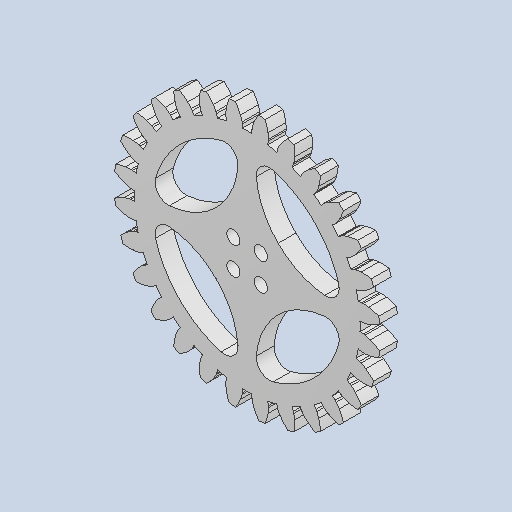
# Autodesk Inventor part: 最終段m2z28t4
Saved by Autodesk Inventor 2023 (Build 270158030, 158C)
## iProperties
Created: 2022-01-10
Part Number: 最終段m2z28t4
Material: Aluminum 2014-T6
Document SubType Name: Modeling
Designer: acps
Density: 2.78927 g/cm^3
Appearance: Satin
Author: acps
Autodesk Inventor part; units mm, degrees
ref_plane "YZ Plane" through (0, 0, 0) normal (1, 0, 0) x (0, 1, 0)
ref_plane "XZ Plane" through (0, 0, 0) normal (0, 1, 0) x (-1, 0, 0)
ref_plane "XY Plane" through (0, 0, 0) normal (0, 0, 1) x (1, 0, 0)
sketch "Sketch1" plane through (0, 0, 0) normal (0, 0, 1) x (1, 0, 0)
  arc A0 (1.1408, 26.6584) -> (1.0836, 26.2891) centre (3.5659, 26.0938) ccw
  arc A1 (1.5089, 27.8103) -> (1.1408, 26.6584) centre (7.8128, 25.1608) ccw
  arc A2 (2.6316, 29.8844) -> (1.5089, 27.8103) centre (12.3866, 23.2633) ccw
  arc A3 (-4.8199, 26.2439) -> (-4.7934, 25.8711) centre (-2.3299, 26.2331) ccw
  arc A4 (-4.7173, 27.4488) -> (-4.8199, 26.2439) centre (2.0181, 26.2684) ccw
  arc A5 (-4.0843, 29.7207) -> (-4.7173, 27.4488) centre (6.8995, 25.4363) ccw
  arc A6 (-10.5388, 24.5133) -> (-10.4301, 24.1558) centre (-8.1089, 25.0569) ccw
  arc A7 (-10.7069, 25.7109) -> (-10.5388, 24.5133) centre (-3.8778, 26.0589) ccw
  arc A8 (-10.5954, 28.0667) -> (-10.7069, 25.7109) centre (1.0664, 26.3339) ccw
  arc A9 (-15.7293, 21.5536) -> (-15.5438, 21.2292) centre (-13.4813, 22.6243) ccw
  arc A10 (-16.1597, 22.6838) -> (-15.7293, 21.5536) centre (-9.5792, 24.5427) ccw
  arc A11 (-16.5751, 25.0053) -> (-16.1597, 22.6838) centre (-4.8202, 25.9109) ccw
  arc A12 (-20.1311, 17.5131) -> (-19.878, 17.2382) centre (-18.1776, 19.0572) ccw
  arc A13 (-20.8022, 18.5192) -> (-20.1311, 17.5131) centre (-14.8003, 21.7958) ccw
  arc A14 (-21.7238, 20.69) -> (-20.8022, 18.5192) centre (-10.4651, 24.1887) ccw
  arc A15 (-23.5234, 12.5944) -> (-23.2155, 12.3827) centre (-21.9625, 14.5345) ccw
  arc A16 (-24.4015, 13.4259) -> (-23.5234, 12.5944) centre (-19.2792, 17.9559) ccw
  arc A17 (-25.7831, 15.3373) -> (-24.4015, 13.4259) centre (-15.5852, 21.2535) ccw
  arc A18 (-25.7362, 7.0442) -> (-25.3888, 6.9063) centre (-24.6461, 9.283) ccw
  arc A19 (-26.7773, 7.6595) -> (-25.7362, 7.0442) centre (-22.7914, 13.2157) ccw
  arc A20 (-28.5495, 9.2155) -> (-26.7773, 7.6595) centre (-19.9238, 17.2526) ccw
  arc A21 (-26.6584, 1.1408) -> (-26.2891, 1.0836) centre (-26.0938, 3.5659) ccw
  arc A22 (-27.8103, 1.5089) -> (-26.6584, 1.1408) centre (-25.1608, 7.8128) ccw
  arc A23 (-29.8844, 2.6316) -> (-27.8103, 1.5089) centre (-23.2633, 12.3866) ccw
  arc A24 (-26.2439, -4.8199) -> (-25.8711, -4.7934) centre (-26.2331, -2.3299) ccw
  arc A25 (-27.4488, -4.7173) -> (-26.2439, -4.8199) centre (-26.2684, 2.0181) ccw
  arc A26 (-29.7207, -4.0843) -> (-27.4488, -4.7173) centre (-25.4363, 6.8995) ccw
  arc A27 (-24.5133, -10.5388) -> (-24.1558, -10.4301) centre (-25.0569, -8.1089) ccw
  arc A28 (-25.7109, -10.7069) -> (-24.5133, -10.5388) centre (-26.0589, -3.8778) ccw
  arc A29 (-28.0667, -10.5954) -> (-25.7109, -10.7069) centre (-26.3339, 1.0664) ccw
  arc A30 (-21.5536, -15.7293) -> (-21.2292, -15.5438) centre (-22.6243, -13.4813) ccw
  arc A31 (-22.6838, -16.1597) -> (-21.5536, -15.7293) centre (-24.5427, -9.5792) ccw
  arc A32 (-25.0053, -16.5751) -> (-22.6838, -16.1597) centre (-25.9109, -4.8202) ccw
  arc A33 (-17.5131, -20.1311) -> (-17.2382, -19.878) centre (-19.0572, -18.1776) ccw
  arc A34 (-18.5192, -20.8022) -> (-17.5131, -20.1311) centre (-21.7958, -14.8003) ccw
  arc A35 (-20.69, -21.7238) -> (-18.5192, -20.8022) centre (-24.1887, -10.4651) ccw
  arc A36 (-12.5944, -23.5234) -> (-12.3827, -23.2155) centre (-14.5345, -21.9625) ccw
  arc A37 (-13.4259, -24.4015) -> (-12.5944, -23.5234) centre (-17.9559, -19.2792) ccw
  arc A38 (-15.3373, -25.7831) -> (-13.4259, -24.4015) centre (-21.2535, -15.5852) ccw
  arc A39 (-7.0442, -25.7362) -> (-6.9063, -25.3888) centre (-9.283, -24.6461) ccw
  arc A40 (-7.6595, -26.7773) -> (-7.0442, -25.7362) centre (-13.2157, -22.7914) ccw
  arc A41 (-9.2155, -28.5495) -> (-7.6595, -26.7773) centre (-17.2526, -19.9238) ccw
  arc A42 (-1.1408, -26.6584) -> (-1.0836, -26.2891) centre (-3.5659, -26.0938) ccw
  arc A43 (-1.5089, -27.8103) -> (-1.1408, -26.6584) centre (-7.8128, -25.1608) ccw
  arc A44 (-2.6316, -29.8844) -> (-1.5089, -27.8103) centre (-12.3866, -23.2633) ccw
  arc A45 (4.8199, -26.2439) -> (4.7934, -25.8711) centre (2.3299, -26.2331) ccw
  arc A46 (4.7173, -27.4488) -> (4.8199, -26.2439) centre (-2.0181, -26.2684) ccw
  arc A47 (4.0843, -29.7207) -> (4.7173, -27.4488) centre (-6.8995, -25.4363) ccw
  arc A48 (10.5388, -24.5133) -> (10.4301, -24.1558) centre (8.1089, -25.0569) ccw
  arc A49 (10.7069, -25.7109) -> (10.5388, -24.5133) centre (3.8778, -26.0589) ccw
  arc A50 (10.5954, -28.0667) -> (10.7069, -25.7109) centre (-1.0664, -26.3339) ccw
  arc A51 (15.7293, -21.5536) -> (15.5438, -21.2292) centre (13.4813, -22.6243) ccw
  arc A52 (16.1597, -22.6838) -> (15.7293, -21.5536) centre (9.5792, -24.5427) ccw
  arc A53 (16.5751, -25.0053) -> (16.1597, -22.6838) centre (4.8202, -25.9109) ccw
  arc A54 (20.1311, -17.5131) -> (19.878, -17.2382) centre (18.1776, -19.0572) ccw
  arc A55 (20.8022, -18.5192) -> (20.1311, -17.5131) centre (14.8003, -21.7958) ccw
  arc A56 (21.7238, -20.69) -> (20.8022, -18.5192) centre (10.4651, -24.1887) ccw
  arc A57 (23.5234, -12.5944) -> (23.2155, -12.3827) centre (21.9625, -14.5345) ccw
  arc A58 (24.4015, -13.4259) -> (23.5234, -12.5944) centre (19.2792, -17.9559) ccw
  arc A59 (25.7831, -15.3373) -> (24.4015, -13.4259) centre (15.5852, -21.2535) ccw
  arc A60 (25.7362, -7.0442) -> (25.3888, -6.9063) centre (24.6461, -9.283) ccw
  arc A61 (26.7773, -7.6595) -> (25.7362, -7.0442) centre (22.7914, -13.2157) ccw
  arc A62 (28.5495, -9.2155) -> (26.7773, -7.6595) centre (19.9238, -17.2526) ccw
  arc A63 (26.6584, -1.1408) -> (26.2891, -1.0836) centre (26.0938, -3.5659) ccw
  arc A64 (27.8103, -1.5089) -> (26.6584, -1.1408) centre (25.1608, -7.8128) ccw
  arc A65 (29.8844, -2.6316) -> (27.8103, -1.5089) centre (23.2633, -12.3866) ccw
  arc A66 (26.2439, 4.8199) -> (25.8711, 4.7934) centre (26.2331, 2.3299) ccw
  arc A67 (27.4488, 4.7173) -> (26.2439, 4.8199) centre (26.2684, -2.0181) ccw
  arc A68 (29.7207, 4.0843) -> (27.4488, 4.7173) centre (25.4363, -6.8995) ccw
  arc A69 (24.5133, 10.5388) -> (24.1558, 10.4301) centre (25.0569, 8.1089) ccw
  arc A70 (25.7109, 10.7069) -> (24.5133, 10.5388) centre (26.0589, 3.8778) ccw
  arc A71 (28.0667, 10.5954) -> (25.7109, 10.7069) centre (26.3339, -1.0664) ccw
  arc A72 (21.5536, 15.7293) -> (21.2292, 15.5438) centre (22.6243, 13.4813) ccw
  arc A73 (22.6838, 16.1597) -> (21.5536, 15.7293) centre (24.5427, 9.5792) ccw
  arc A74 (25.0053, 16.5751) -> (22.6838, 16.1597) centre (25.9109, 4.8202) ccw
  arc A75 (17.5131, 20.1311) -> (17.2382, 19.878) centre (19.0572, 18.1776) ccw
  arc A76 (18.5192, 20.8022) -> (17.5131, 20.1311) centre (21.7958, 14.8003) ccw
  arc A77 (20.69, 21.7238) -> (18.5192, 20.8022) centre (24.1887, 10.4651) ccw
  arc A78 (12.5944, 23.5234) -> (12.3827, 23.2155) centre (14.5345, 21.9625) ccw
  arc A79 (13.4259, 24.4015) -> (12.5944, 23.5234) centre (17.9559, 19.2792) ccw
  arc A80 (15.3373, 25.7831) -> (13.4259, 24.4015) centre (21.2535, 15.5852) ccw
  arc A81 (7.0442, 25.7362) -> (6.9063, 25.3888) centre (9.283, 24.6461) ccw
  arc A82 (7.6595, 26.7773) -> (7.0442, 25.7362) centre (13.2157, 22.7914) ccw
  arc A83 (9.2155, 28.5495) -> (7.6595, 26.7773) centre (17.2526, 19.9238) ccw
  arc A84 (-1.0836, 26.2891) -> (-1.1408, 26.6584) centre (-3.5659, 26.0938) ccw
  arc A85 (-1.1408, 26.6584) -> (-1.5089, 27.8103) centre (-7.8128, 25.1608) ccw
  arc A86 (-1.5089, 27.8103) -> (-2.6316, 29.8844) centre (-12.3866, 23.2633) ccw
  arc A87 (-6.9063, 25.3888) -> (-7.0442, 25.7362) centre (-9.283, 24.6461) ccw
  arc A88 (-7.0442, 25.7362) -> (-7.6595, 26.7773) centre (-13.2157, 22.7914) ccw
  arc A89 (-7.6595, 26.7773) -> (-9.2155, 28.5495) centre (-17.2526, 19.9238) ccw
  arc A90 (-12.3827, 23.2155) -> (-12.5944, 23.5234) centre (-14.5345, 21.9625) ccw
  arc A91 (-12.5944, 23.5234) -> (-13.4259, 24.4015) centre (-17.9559, 19.2792) ccw
  arc A92 (-13.4259, 24.4015) -> (-15.3373, 25.7831) centre (-21.2535, 15.5852) ccw
  arc A93 (-17.2382, 19.878) -> (-17.5131, 20.1311) centre (-19.0572, 18.1776) ccw
  arc A94 (-17.5131, 20.1311) -> (-18.5192, 20.8022) centre (-21.7958, 14.8003) ccw
  arc A95 (-18.5192, 20.8022) -> (-20.69, 21.7238) centre (-24.1887, 10.4651) ccw
  arc A96 (-21.2292, 15.5438) -> (-21.5536, 15.7293) centre (-22.6243, 13.4813) ccw
  arc A97 (-21.5536, 15.7293) -> (-22.6838, 16.1597) centre (-24.5427, 9.5792) ccw
  arc A98 (-22.6838, 16.1597) -> (-25.0053, 16.5751) centre (-25.9109, 4.8202) ccw
  arc A99 (-24.1558, 10.4301) -> (-24.5133, 10.5388) centre (-25.0569, 8.1089) ccw
  arc A100 (-24.5133, 10.5388) -> (-25.7109, 10.7069) centre (-26.0589, 3.8778) ccw
  arc A101 (-25.7109, 10.7069) -> (-28.0667, 10.5954) centre (-26.3339, -1.0664) ccw
  arc A102 (-25.8711, 4.7934) -> (-26.2439, 4.8199) centre (-26.2331, 2.3299) ccw
  arc A103 (-26.2439, 4.8199) -> (-27.4488, 4.7173) centre (-26.2684, -2.0181) ccw
  arc A104 (-27.4488, 4.7173) -> (-29.7207, 4.0843) centre (-25.4363, -6.8995) ccw
  arc A105 (-26.2891, -1.0836) -> (-26.6584, -1.1408) centre (-26.0938, -3.5659) ccw
  arc A106 (-26.6584, -1.1408) -> (-27.8103, -1.5089) centre (-25.1608, -7.8128) ccw
  arc A107 (-27.8103, -1.5089) -> (-29.8844, -2.6316) centre (-23.2633, -12.3866) ccw
  arc A108 (-25.3888, -6.9063) -> (-25.7362, -7.0442) centre (-24.6461, -9.283) ccw
  arc A109 (-25.7362, -7.0442) -> (-26.7773, -7.6595) centre (-22.7914, -13.2157) ccw
  arc A110 (-26.7773, -7.6595) -> (-28.5495, -9.2155) centre (-19.9238, -17.2526) ccw
  arc A111 (-23.2155, -12.3827) -> (-23.5234, -12.5944) centre (-21.9625, -14.5345) ccw
  arc A112 (-23.5234, -12.5944) -> (-24.4015, -13.4259) centre (-19.2792, -17.9559) ccw
  arc A113 (-24.4015, -13.4259) -> (-25.7831, -15.3373) centre (-15.5852, -21.2535) ccw
  arc A114 (-19.878, -17.2382) -> (-20.1311, -17.5131) centre (-18.1776, -19.0572) ccw
  arc A115 (-20.1311, -17.5131) -> (-20.8022, -18.5192) centre (-14.8003, -21.7958) ccw
  arc A116 (-20.8022, -18.5192) -> (-21.7238, -20.69) centre (-10.4651, -24.1887) ccw
  arc A117 (-15.5438, -21.2292) -> (-15.7293, -21.5536) centre (-13.4813, -22.6243) ccw
  arc A118 (-15.7293, -21.5536) -> (-16.1597, -22.6838) centre (-9.5792, -24.5427) ccw
  arc A119 (-16.1597, -22.6838) -> (-16.5751, -25.0053) centre (-4.8202, -25.9109) ccw
  arc A120 (-10.4301, -24.1558) -> (-10.5388, -24.5133) centre (-8.1089, -25.0569) ccw
  arc A121 (-10.5388, -24.5133) -> (-10.7069, -25.7109) centre (-3.8778, -26.0589) ccw
  arc A122 (-10.7069, -25.7109) -> (-10.5954, -28.0667) centre (1.0664, -26.3339) ccw
  arc A123 (-4.7934, -25.8711) -> (-4.8199, -26.2439) centre (-2.3299, -26.2331) ccw
  arc A124 (-4.8199, -26.2439) -> (-4.7173, -27.4488) centre (2.0181, -26.2684) ccw
  arc A125 (-4.7173, -27.4488) -> (-4.0843, -29.7207) centre (6.8995, -25.4363) ccw
  arc A126 (1.0836, -26.2891) -> (1.1408, -26.6584) centre (3.5659, -26.0938) ccw
  arc A127 (1.1408, -26.6584) -> (1.5089, -27.8103) centre (7.8128, -25.1608) ccw
  arc A128 (1.5089, -27.8103) -> (2.6316, -29.8844) centre (12.3866, -23.2633) ccw
  arc A129 (6.9063, -25.3888) -> (7.0442, -25.7362) centre (9.283, -24.6461) ccw
  arc A130 (7.0442, -25.7362) -> (7.6595, -26.7773) centre (13.2157, -22.7914) ccw
  arc A131 (7.6595, -26.7773) -> (9.2155, -28.5495) centre (17.2526, -19.9238) ccw
  arc A132 (12.3827, -23.2155) -> (12.5944, -23.5234) centre (14.5345, -21.9625) ccw
  arc A133 (12.5944, -23.5234) -> (13.4259, -24.4015) centre (17.9559, -19.2792) ccw
  arc A134 (13.4259, -24.4015) -> (15.3373, -25.7831) centre (21.2535, -15.5852) ccw
  arc A135 (17.2382, -19.878) -> (17.5131, -20.1311) centre (19.0572, -18.1776) ccw
  arc A136 (17.5131, -20.1311) -> (18.5192, -20.8022) centre (21.7958, -14.8003) ccw
  arc A137 (18.5192, -20.8022) -> (20.69, -21.7238) centre (24.1887, -10.4651) ccw
  arc A138 (21.2292, -15.5438) -> (21.5536, -15.7293) centre (22.6243, -13.4813) ccw
  arc A139 (21.5536, -15.7293) -> (22.6838, -16.1597) centre (24.5427, -9.5792) ccw
  arc A140 (22.6838, -16.1597) -> (25.0053, -16.5751) centre (25.9109, -4.8202) ccw
  arc A141 (24.1558, -10.4301) -> (24.5133, -10.5388) centre (25.0569, -8.1089) ccw
  arc A142 (24.5133, -10.5388) -> (25.7109, -10.7069) centre (26.0589, -3.8778) ccw
  arc A143 (25.7109, -10.7069) -> (28.0667, -10.5954) centre (26.3339, 1.0664) ccw
  arc A144 (25.8711, -4.7934) -> (26.2439, -4.8199) centre (26.2331, -2.3299) ccw
  arc A145 (26.2439, -4.8199) -> (27.4488, -4.7173) centre (26.2684, 2.0181) ccw
  arc A146 (27.4488, -4.7173) -> (29.7207, -4.0843) centre (25.4363, 6.8995) ccw
  arc A147 (26.2891, 1.0836) -> (26.6584, 1.1408) centre (26.0938, 3.5659) ccw
  arc A148 (26.6584, 1.1408) -> (27.8103, 1.5089) centre (25.1608, 7.8128) ccw
  arc A149 (27.8103, 1.5089) -> (29.8844, 2.6316) centre (23.2633, 12.3866) ccw
  arc A150 (25.3888, 6.9063) -> (25.7362, 7.0442) centre (24.6461, 9.283) ccw
  arc A151 (25.7362, 7.0442) -> (26.7773, 7.6595) centre (22.7914, 13.2157) ccw
  arc A152 (26.7773, 7.6595) -> (28.5495, 9.2155) centre (19.9238, 17.2526) ccw
  arc A153 (23.2155, 12.3827) -> (23.5234, 12.5944) centre (21.9625, 14.5345) ccw
  arc A154 (23.5234, 12.5944) -> (24.4015, 13.4259) centre (19.2792, 17.9559) ccw
  arc A155 (24.4015, 13.4259) -> (25.7831, 15.3373) centre (15.5852, 21.2535) ccw
  arc A156 (19.878, 17.2382) -> (20.1311, 17.5131) centre (18.1776, 19.0572) ccw
  arc A157 (20.1311, 17.5131) -> (20.8022, 18.5192) centre (14.8003, 21.7958) ccw
  arc A158 (20.8022, 18.5192) -> (21.7238, 20.69) centre (10.4651, 24.1887) ccw
  arc A159 (15.5438, 21.2292) -> (15.7293, 21.5536) centre (13.4813, 22.6243) ccw
  arc A160 (15.7293, 21.5536) -> (16.1597, 22.6838) centre (9.5792, 24.5427) ccw
  arc A161 (16.1597, 22.6838) -> (16.5751, 25.0053) centre (4.8202, 25.9109) ccw
  arc A162 (10.4301, 24.1558) -> (10.5388, 24.5133) centre (8.1089, 25.0569) ccw
  arc A163 (10.5388, 24.5133) -> (10.7069, 25.7109) centre (3.8778, 26.0589) ccw
  arc A164 (10.7069, 25.7109) -> (10.5954, 28.0667) centre (-1.0664, 26.3339) ccw
  arc A165 (4.7934, 25.8711) -> (4.8199, 26.2439) centre (2.3299, 26.2331) ccw
  arc A166 (4.8199, 26.2439) -> (4.7173, 27.4488) centre (-2.0181, 26.2684) ccw
  arc A167 (4.7173, 27.4488) -> (4.0843, 29.7207) centre (-6.8995, 25.4363) ccw
  arc A168 (1.0502, 25.4784) -> (-1.0502, 25.4784) centre (0, 0) ccw
  arc A169 (-4.6456, 25.0733) -> (-6.6933, 24.6059) centre (0, 0) ccw
  arc A170 (-10.1085, 23.4109) -> (-12.0008, 22.4996) centre (0, 0) ccw
  arc A171 (-15.0644, 20.5746) -> (-16.7066, 19.265) centre (0, 0) ccw
  arc A172 (-19.265, 16.7066) -> (-20.5746, 15.0644) centre (0, 0) ccw
  arc A173 (-22.4996, 12.0008) -> (-23.4109, 10.1085) centre (0, 0) ccw
  arc A174 (-24.6059, 6.6933) -> (-25.0733, 4.6456) centre (0, 0) ccw
  arc A175 (-25.4784, 1.0502) -> (-25.4784, -1.0502) centre (0, 0) ccw
  arc A176 (-25.0733, -4.6456) -> (-24.6059, -6.6933) centre (0, 0) ccw
  arc A177 (-23.4109, -10.1085) -> (-22.4996, -12.0008) centre (0, 0) ccw
  arc A178 (-20.5746, -15.0644) -> (-19.265, -16.7066) centre (0, 0) ccw
  arc A179 (-16.7066, -19.265) -> (-15.0644, -20.5746) centre (0, 0) ccw
  arc A180 (-12.0008, -22.4996) -> (-10.1085, -23.4109) centre (0, 0) ccw
  arc A181 (-6.6933, -24.6059) -> (-4.6456, -25.0733) centre (0, 0) ccw
  arc A182 (-1.0502, -25.4784) -> (1.0502, -25.4784) centre (0, 0) ccw
  arc A183 (4.6456, -25.0733) -> (6.6933, -24.6059) centre (0, 0) ccw
  arc A184 (10.1085, -23.4109) -> (12.0008, -22.4996) centre (0, 0) ccw
  arc A185 (15.0644, -20.5746) -> (16.7066, -19.265) centre (0, 0) ccw
  arc A186 (19.265, -16.7066) -> (20.5746, -15.0644) centre (0, 0) ccw
  arc A187 (22.4996, -12.0008) -> (23.4109, -10.1085) centre (0, 0) ccw
  arc A188 (24.6059, -6.6933) -> (25.0733, -4.6456) centre (0, 0) ccw
  arc A189 (25.4784, -1.0502) -> (25.4784, 1.0502) centre (0, 0) ccw
  arc A190 (25.0733, 4.6456) -> (24.6059, 6.6933) centre (0, 0) ccw
  arc A191 (23.4109, 10.1085) -> (22.4996, 12.0008) centre (0, 0) ccw
  arc A192 (20.5746, 15.0644) -> (19.265, 16.7066) centre (0, 0) ccw
  arc A193 (16.7066, 19.265) -> (15.0644, 20.5746) centre (0, 0) ccw
  arc A194 (12.0008, 22.4996) -> (10.1085, 23.4109) centre (0, 0) ccw
  arc A195 (6.6933, 24.6059) -> (4.6456, 25.0733) centre (0, 0) ccw
  arc A196 (-2.6316, 29.8844) -> (-4.0843, 29.7207) centre (0, 0) ccw
  arc A197 (-9.2155, 28.5495) -> (-10.5954, 28.0667) centre (0, 0) ccw
  arc A198 (-15.3373, 25.7831) -> (-16.5751, 25.0053) centre (0, 0) ccw
  arc A199 (-20.69, 21.7238) -> (-21.7238, 20.69) centre (0, 0) ccw
  arc A200 (-25.0053, 16.5751) -> (-25.7831, 15.3373) centre (0, 0) ccw
  arc A201 (-28.0667, 10.5954) -> (-28.5495, 9.2155) centre (0, 0) ccw
  arc A202 (-29.7207, 4.0843) -> (-29.8844, 2.6316) centre (0, 0) ccw
  arc A203 (-29.8844, -2.6316) -> (-29.7207, -4.0843) centre (0, 0) ccw
  arc A204 (-28.5495, -9.2155) -> (-28.0667, -10.5954) centre (0, 0) ccw
  arc A205 (-25.7831, -15.3373) -> (-25.0053, -16.5751) centre (0, 0) ccw
  arc A206 (-21.7238, -20.69) -> (-20.69, -21.7238) centre (0, 0) ccw
  arc A207 (-16.5751, -25.0053) -> (-15.3373, -25.7831) centre (0, 0) ccw
  arc A208 (-10.5954, -28.0667) -> (-9.2155, -28.5495) centre (0, 0) ccw
  arc A209 (-4.0843, -29.7207) -> (-2.6316, -29.8844) centre (0, 0) ccw
  arc A210 (2.6316, -29.8844) -> (4.0843, -29.7207) centre (0, 0) ccw
  arc A211 (9.2155, -28.5495) -> (10.5954, -28.0667) centre (0, 0) ccw
  arc A212 (15.3373, -25.7831) -> (16.5751, -25.0053) centre (0, 0) ccw
  arc A213 (20.69, -21.7238) -> (21.7238, -20.69) centre (0, 0) ccw
  arc A214 (25.0053, -16.5751) -> (25.7831, -15.3373) centre (0, 0) ccw
  arc A215 (28.0667, -10.5954) -> (28.5495, -9.2155) centre (0, 0) ccw
  arc A216 (29.7207, -4.0843) -> (29.8844, -2.6316) centre (0, 0) ccw
  arc A217 (29.8844, 2.6316) -> (29.7207, 4.0843) centre (0, 0) ccw
  arc A218 (28.5495, 9.2155) -> (28.0667, 10.5954) centre (0, 0) ccw
  arc A219 (25.7831, 15.3373) -> (25.0053, 16.5751) centre (0, 0) ccw
  arc A220 (21.7238, 20.69) -> (20.69, 21.7238) centre (0, 0) ccw
  arc A221 (16.5751, 25.0053) -> (15.3373, 25.7831) centre (0, 0) ccw
  arc A222 (10.5954, 28.0667) -> (9.2155, 28.5495) centre (0, 0) ccw
  arc A223 (4.0843, 29.7207) -> (2.6316, 29.8844) centre (0, 0) ccw
  line L0 (1.0502, 25.4784) -> (1.0836, 26.2891)
  line L1 (-4.6456, 25.0733) -> (-4.7934, 25.8711)
  line L2 (-10.1085, 23.4109) -> (-10.4301, 24.1558)
  line L3 (-15.0644, 20.5746) -> (-15.5438, 21.2292)
  line L4 (-19.265, 16.7066) -> (-19.878, 17.2382)
  line L5 (-22.4996, 12.0008) -> (-23.2155, 12.3827)
  line L6 (-24.6059, 6.6933) -> (-25.3888, 6.9063)
  line L7 (-25.4784, 1.0502) -> (-26.2891, 1.0836)
  line L8 (-25.0733, -4.6456) -> (-25.8711, -4.7934)
  line L9 (-23.4109, -10.1085) -> (-24.1558, -10.4301)
  line L10 (-20.5746, -15.0644) -> (-21.2292, -15.5438)
  line L11 (-16.7066, -19.265) -> (-17.2382, -19.878)
  line L12 (-12.0008, -22.4996) -> (-12.3827, -23.2155)
  line L13 (-6.6933, -24.6059) -> (-6.9063, -25.3888)
  line L14 (-1.0502, -25.4784) -> (-1.0836, -26.2891)
  line L15 (4.6456, -25.0733) -> (4.7934, -25.8711)
  line L16 (10.1085, -23.4109) -> (10.4301, -24.1558)
  line L17 (15.0644, -20.5746) -> (15.5438, -21.2292)
  line L18 (19.265, -16.7066) -> (19.878, -17.2382)
  line L19 (22.4996, -12.0008) -> (23.2155, -12.3827)
  line L20 (24.6059, -6.6933) -> (25.3888, -6.9063)
  line L21 (25.4784, -1.0502) -> (26.2891, -1.0836)
  line L22 (25.0733, 4.6456) -> (25.8711, 4.7934)
  line L23 (23.4109, 10.1085) -> (24.1558, 10.4301)
  line L24 (20.5746, 15.0644) -> (21.2292, 15.5438)
  line L25 (16.7066, 19.265) -> (17.2382, 19.878)
  line L26 (12.0008, 22.4996) -> (12.3827, 23.2155)
  line L27 (6.6933, 24.6059) -> (6.9063, 25.3888)
  line L28 (-1.0502, 25.4784) -> (-1.0836, 26.2891)
  line L29 (-6.6933, 24.6059) -> (-6.9063, 25.3888)
  line L30 (-12.0008, 22.4996) -> (-12.3827, 23.2155)
  line L31 (-16.7066, 19.265) -> (-17.2382, 19.878)
  line L32 (-20.5746, 15.0644) -> (-21.2292, 15.5438)
  line L33 (-23.4109, 10.1085) -> (-24.1558, 10.4301)
  line L34 (-25.0733, 4.6456) -> (-25.8711, 4.7934)
  line L35 (-25.4784, -1.0502) -> (-26.2891, -1.0836)
  line L36 (-24.6059, -6.6933) -> (-25.3888, -6.9063)
  line L37 (-22.4996, -12.0008) -> (-23.2155, -12.3827)
  line L38 (-19.265, -16.7066) -> (-19.878, -17.2382)
  line L39 (-15.0644, -20.5746) -> (-15.5438, -21.2292)
  line L40 (-10.1085, -23.4109) -> (-10.4301, -24.1558)
  line L41 (-4.6456, -25.0733) -> (-4.7934, -25.8711)
  line L42 (1.0502, -25.4784) -> (1.0836, -26.2891)
  line L43 (6.6933, -24.6059) -> (6.9063, -25.3888)
  line L44 (12.0008, -22.4996) -> (12.3827, -23.2155)
  line L45 (16.7066, -19.265) -> (17.2382, -19.878)
  line L46 (20.5746, -15.0644) -> (21.2292, -15.5438)
  line L47 (23.4109, -10.1085) -> (24.1558, -10.4301)
  line L48 (25.0733, -4.6456) -> (25.8711, -4.7934)
  line L49 (25.4784, 1.0502) -> (26.2891, 1.0836)
  line L50 (24.6059, 6.6933) -> (25.3888, 6.9063)
  line L51 (22.4996, 12.0008) -> (23.2155, 12.3827)
  line L52 (19.265, 16.7066) -> (19.878, 17.2382)
  line L53 (15.0644, 20.5746) -> (15.5438, 21.2292)
  line L54 (10.1085, 23.4109) -> (10.4301, 24.1558)
  line L55 (4.6456, 25.0733) -> (4.7934, 25.8711)
  point P0 (0, 0)
  constraints: 336 point on circle, 168 centre point, 112 end point, 2 horizontal alignment, 2 vertical alignment, 164 other
extrude "Extrusion1" add sketch "Sketch1" along normal blind 4
sketch "Sketch2" plane through (0, 0, 4) normal (0, 0, 1) x (1, 0, 0)
  circle A0 centre (-3.1, 3.1) radius 1.5
  circle A1 centre (-3.1, -3.1) radius 1.5
  circle A2 centre (3.1, -3.1) radius 1.5
  circle A3 centre (3.1, 3.1) radius 1.5
  point P0 (0, 0)
  dimension "d2" = 3
  dimension "d8" = 360
  dimension "d10" = 6.2
  constraints: 4 centre point, 1 horizontal alignment, 9 other
  measures "d2" diameter of A0
  measures "d10" distance of A3.centre A0.centre
extrude "Extrusion2" cut sketch "Sketch2" against normal through all
sketch "Sketch3" plane through (0, 0, 4) normal (0, 0, 1) x (1, 0, 0)
  arc A0 (-15.0644, 20.5746) -> (-16.7066, 19.265) centre (0, 0) ccw projected
  circle A1 centre (0, 0) radius 25.5 construction
  circle A2 centre (0, 0) radius 21.5
  arc A3 (-2.065, 17.5342) -> (-5.8731, 20.6823) centre (-5.0536, 17.7964) ccw
  circle A4 centre (0, 0) radius 5.8841 construction
  circle A5 centre (3.1, 3.1) radius 1.5 projected
  circle A6 centre (0, 0) radius 9.8841
  arc A7 (-6.9854, 6.9927) -> (-2.065, 17.5342) centre (-19, 19.0198) ccw
  line L0 (0, 0) -> (0, 11.6047) construction
  arc A8 (5.8731, 20.6823) -> (2.065, 17.5342) centre (5.0536, 17.7964) ccw
  arc A9 (2.065, 17.5342) -> (6.9854, 6.9927) centre (19, 19.0198) ccw
  arc A10 (-17.5342, 2.065) -> (-6.9927, 6.9854) centre (-19.0198, 19) ccw
  arc A11 (-20.6823, 5.8731) -> (-17.5342, 2.065) centre (-17.7964, 5.0536) ccw
  arc A12 (-17.5342, -2.065) -> (-20.6823, -5.8731) centre (-17.7964, -5.0536) ccw
  arc A13 (-6.9927, -6.9854) -> (-17.5342, -2.065) centre (-19.0198, -19) ccw
  arc A14 (-2.065, -17.5342) -> (-6.9854, -6.9927) centre (-19, -19.0198) ccw
  arc A15 (-5.8731, -20.6823) -> (-2.065, -17.5342) centre (-5.0536, -17.7964) ccw
  arc A16 (2.065, -17.5342) -> (5.8731, -20.6823) centre (5.0536, -17.7964) ccw
  arc A17 (6.9854, -6.9927) -> (2.065, -17.5342) centre (19, -19.0198) ccw
  arc A18 (17.5342, -2.065) -> (6.9927, -6.9854) centre (19.0198, -19) ccw
  arc A19 (20.6823, -5.8731) -> (17.5342, -2.065) centre (17.7964, -5.0536) ccw
  arc A20 (17.5342, 2.065) -> (20.6823, 5.8731) centre (17.7964, 5.0536) ccw
  arc A21 (6.9927, 6.9854) -> (17.5342, 2.065) centre (19.0198, 19) ccw
  point P0 (0, 0)
  point P1 (20.6823, -5.8731)
  point P2 (6.9927, -6.9854)
  point P3 (5.8731, -20.6823)
  point P4 (-5.8731, -20.6823)
  point P5 (-6.9854, -6.9927)
  point P6 (-6.9927, -6.9854)
  point P7 (-20.6823, -5.8731)
  point P8 (-20.6823, 5.8731)
  point P9 (-6.9927, 6.9854)
  point P10 (20.6823, 5.8731)
  point P11 (5.8731, 20.6823)
  point P12 (6.9854, 6.9927)
  dimension "d13" = 4
  dimension "d14" = 3
  dimension "d16" = 4
  dimension "d17" = 17
  dimension "d18" = 19
  dimension "d21" = 360
  constraints: 32 point on circle, 18 centre point, 5 symmetric about line, 2 coincident, 2 end point, 2 tangent, 1 concentric, 1 vertical, 67 other
  measures "d14" radius of A3
  measures "d17" radius of A7
  measures "d18" distance from line of L0 A7.centre
extrude "Extrusion3" cut sketch "Sketch3" against normal through all contours A20 A21 A6 A9 A8 A2 | A2 A16 A17 A6 A18 A19 | A3 A7 A6 A10 A11 A2 | A2 A12 A13 A6 A14 A15
body "Solid1"
